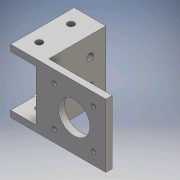
# Autodesk Inventor part: Part1
Saved by Autodesk Inventor 2016 (Build 200138000, 138)
## iProperties
Created: 2015-11-15
Part Number: Part1
Material: Generic
Document SubType Name: Modeling
Designer: Solomon
Density: 1 g/cm^3
Appearance: Default
Author: Solomon
Autodesk Inventor part; units mm, degrees
ref_plane "YZ Plane" through (0, 0, 0) normal (1, 0, 0) x (0, 1, 0)
ref_plane "XZ Plane" through (0, 0, 0) normal (0, 1, 0) x (-1, 0, 0)
ref_plane "XY Plane" through (0, 0, 0) normal (0, 0, 1) x (1, 0, 0)
sketch "Sketch1" plane through (0, 0, 0) normal (0, 1, 0) x (-1, 0, 0)
  line L0 (13.85, 15.5) -> (-13.85, 15.5)
  line L1 (-15.5, 13.85) -> (-15.5, -13.85)
  line L2 (-13.85, -15.5) -> (13.85, -15.5)
  line L3 (15.5, -13.85) -> (15.5, 13.85)
  line L4 (15.5, 15.5) -> (-15.5, -15.5) construction
  line L5 (-15.5, 15.5) -> (15.5, -15.5) construction
  circle A0 centre (15.5, 15.5) radius 1.65
  circle A1 centre (15.5, -15.5) radius 1.65
  circle A2 centre (-15.5, 15.5) radius 1.65
  circle A3 centre (-15.5, -15.5) radius 1.65
  line L6 (25, 25) -> (-25, 25)
  line L7 (-25, 25) -> (-25, -25)
  line L8 (-25, -25) -> (25, -25)
  line L9 (25, -25) -> (25, 25)
  line L10 (25, 25) -> (-25, -25) construction
  line L11 (-25, 25) -> (25, -25) construction
  circle A4 centre (0, 0) radius 12.5
  dimension "d2" = 3.3
  dimension "d3" = 3.3
  dimension "d4" = 3.3
  dimension "d5" = 3.3
  dimension "d6" = 27.7
  dimension "d7" = 27.7
  dimension "d8" = 27.7
  dimension "d9" = 27.7
  dimension "d10" = 31
  dimension "d11" = 31
  dimension "d12" = 31
  dimension "d13" = 31
  dimension "d14" = 45
  dimension "d15" = 31
  dimension "d16" = 50
  dimension "d17" = 50
  dimension "d18" = 25
  constraints: 24 end point, 8 point on circle, 5 centre point, 5 coincident, 4 midpoint, 4 parallel, 2 horizontal, 2 perpendicular
  measures "d2" diameter of A0
  measures "d3" diameter of A1
  measures "d4" diameter of A2
  measures "d5" diameter of A3
  measures "d6" distance of L3.start L3.end
  measures "d7" distance of L0.start L0.end
  measures "d8" distance of L2.start L2.end
  measures "d9" distance of L1.start L1.end
  measures "d10" distance of L5.end L4.start
  measures "d11" distance of L4.end L5.end
  measures "d12" distance of L5.start L4.end
  measures "d13" distance of L4.start A2.centre
  measures "d14" angle of L4 L3
  measures "d15" distance between parallel lines of L3 L1
  measures "d16" distance of L8.end L7.end
  measures "d17" distance of L7.end L6.end
  measures "d18" diameter of A4
extrude "Extrusion1" add sketch "Sketch1" along normal blind 5 contours A0 L3 A1 L2 A3 L1 A2 L0 | L9 L8 L7 L6
sketch "Sketch2" plane through (-25, 0, -25) normal (-1, 0, 0) x (0, 0, 1)
  line L0 (0, 0) -> (0, 5) projected
  line L1 (0, 0) -> (50, 0)
  line L2 (50, 0) -> (50, 50)
  line L3 (50, 50) -> (0, 50)
  line L4 (0, 50) -> (0, 0)
  line L5 (25, 50) -> (25, 0)
  line L6 (25, 25) -> (50, 25)
  line L7 (25, 25) -> (0, 25)
  line L8 (25, 25) -> (25, 0)
  line L9 (50, 0) -> (0, 0) projected
  line L10 (25, 12.5) -> (35, 12.5)
  line L11 (25, 12.5) -> (15, 12.5)
  circle A0 centre (35, 12.5) radius 2.65
  circle A1 centre (15, 12.5) radius 2.65
  line L12 (25, 25) -> (25, 50)
  line L13 (25, 37.5) -> (35, 37.5)
  line L14 (25, 37.5) -> (15, 37.5)
  circle A2 centre (15, 37.5) radius 2.65
  circle A3 centre (35, 37.5) radius 2.65
  line L15 (25, 25) -> (25, 0)
  line L16 (12.5, 5) -> (37.5, 5) projected
  line L17 (0, 50) -> (5, 50)
  line L18 (5, 50) -> (5, 0)
  line L19 (5, 0) -> (0, 0)
  line L20 (0, 0) -> (0, 50)
  line L21 (50, 50) -> (45, 50)
  line L22 (45, 50) -> (45, 0)
  line L23 (45, 0) -> (50, 0)
  line L24 (50, 0) -> (50, 50)
  dimension "d21" = 50
  dimension "d22" = 10
  dimension "d23" = 10
  dimension "d24" = 5.3
  dimension "d25" = 5.3
  dimension "d26" = 5.3
  dimension "d27" = 5.3
  dimension "d30" = 5
  dimension "d31" = 5
  constraints: 44 end point, 6 horizontal, 6 midpoint, 6 parallel, 6 perpendicular, 4 centre point, 4 coincident, 2 point on line, 1 collinear, 1 vertical
  measures "d21" distance of L2.end L1.end
  measures "d22" distance of L10.start L10.end
  measures "d23" distance of L10.start L11.end
  measures "d24" diameter of A0
  measures "d25" diameter of A1
  measures "d26" diameter of A2
  measures "d27" diameter of A3
  measures "d30" distance of L18.end L19.end
  measures "d31" distance of L23.end L22.end
extrude "Extrusion2" add sketch "Sketch2" along normal blind 5
sketch "Sketch3" plane through (-30, 0, -25) normal (-1, 0, 0) x (0, 0, 1)
  point P0 (25, 0)
sketch "Sketch4" plane through (-30, 0, -25) normal (-1, 0, 0) x (0, 0, 1)
  line L0 (50, 50) -> (0, 50) projected
  line L1 (0, 0) -> (50, 0) projected
  line L2 (0, 50) -> (5, 50)
  line L3 (5, 50) -> (5, 0)
  line L4 (5, 0) -> (0, 0)
  line L5 (0, 0) -> (0, 50)
  line L6 (50, 5) -> (50, 50) projected
  line L7 (50, 50) -> (45, 50)
  line L8 (45, 50) -> (45, 0)
  line L9 (45, 0) -> (50, 0)
  line L10 (50, 0) -> (50, 50)
  point P0 (25, 0)
  dimension "d32" = 5
  dimension "d33" = 5
  constraints: 16 end point, 4 parallel, 2 horizontal, 2 perpendicular, 2 point on line
  measures "d32" distance of L3.end L4.end
  measures "d33" distance of L9.end L8.end
extrude "Extrusion3" add sketch "Sketch4" along normal blind 20 contours L6 L10 L1 L8 L0 | L3 L1 L5 L0
sketch "Sketch5" plane through (25, 0, -25) normal (0, 0, -1) x (-1, 0, 0)
  line L0 (50, 5) -> (0, 5) projected
  line L1 (75, 50) -> (75, 0) projected
  line L2 (50, 5) -> (75, 5)
  line L3 (75, 5) -> (75, 50)
  line L4 (75, 50) -> (50, 50)
  line L5 (50, 50) -> (50, 5)
  line L6 (50, 5) -> (50, 50) projected
  line L7 (50, 37.5) -> (75, 37.5)
  line L8 (50, 12.5) -> (75, 12.5)
  line L9 (55, 50) -> (55, 0) projected
  line L10 (55, 50) -> (55, 5)
  line L11 (55, 40.15) -> (55, 34.85) projected
  line L12 (55, 37.5) -> (65, 37.5)
  line L13 (55, 15.15) -> (55, 9.85) projected
  line L14 (55, 12.5) -> (65, 12.5)
  circle A0 centre (65, 37.5) radius 2.65
  circle A1 centre (65, 12.5) radius 2.65
  point P0 (25, 0)
  dimension "d36" = 10
  dimension "d37" = 10
  dimension "d38" = 5.3
  dimension "d39" = 5.3
  constraints: 18 end point, 8 point on line, 3 perpendicular, 2 centre point, 2 coincident, 2 midpoint, 2 parallel, 1 horizontal
  measures "d36" distance of L12.start L12.end
  measures "d37" distance of L14.start L14.end
  measures "d38" diameter of A0
  measures "d39" diameter of A1
extrude "Extrusion4" cut sketch "Sketch5" against normal blind 66.25 contours A0 L7 | L7 A0 | A1 L8 | L8 A1
body "Solid1"
